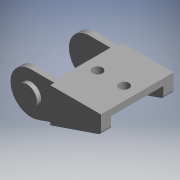
# Autodesk Inventor part: 045-16-2_se08f
Saved by Autodesk Inventor 2017.3 (Build 213256000, 256)
## iProperties
Part Number: 045-16-2_se08f
Material: Generic
Catalog Web Link: www.cadenas.de
Description: 045-16 -1, 045-16-2, 108-_ _-1PZ, 108-_ _-2PZ, 114-_-1PZ, 114-_-2PZ, 117-_-1PZ, 117-_-2PZ, 200F-_-1PZ,200F-_-2PZ, 300F-_-1PZ, 300F-_-2PZ-Flanges for Cable Carriers
Vendor: MISUMI
Document SubType Name: Modeling
Designer: partserver
Manufacturer: MISUMI
Mass: 1.82099 g
Surface Area: 19.911 cm^2
Volume: 1.82099 cm^3
Density: 1 g/cm^3
Appearance: PSOLRGB-192-192-192
Category: PARTsolutions
Company: MISUMI
Title: 045-16-2_se08f
Author: Cadenas PARTsolutions
Comments: Flanges for Cable Carriers
PSOL_IDENT_0: {$CADENAS_DATA\23d-libs\misumi\metric\07_slide_rails\se200f\se08f_body.prj},305 {VTYP=3D},{NB=045-16
PSOL_IDENT_1: -2_se08f},{LINA=045-16-2_se08f},{NN=045-16 -1, 045-16-2, 108-_ _-1PZ, 108-_ _-2PZ, 114-_-1PZ, 114-_-
PSOL_IDENT_2: 2PZ, 117-_-1PZ, 117-_-2PZ, 200F-_-1PZ,200F-_-2PZ, 300F-_-1PZ, 300F-_-2PZ},{DATE=30.06.2021 12:54:06}
PSOL_IDENT_3: ,{GEOMDATE=20.09.2012 00:00:00},{VERSION=},{LINEID=70},{WBVAR=NO,TS},{WBNUMERIC=NO}  {NB=045-16-2_se
PSOL_IDENT_4: 08f},{LINA=045-16-2_se08f},{KT=DUMMY},{PN=045-16-2},{TYPE=045-16},{TYS=045},{NO=16},{TS=2},{MAT=Spec
PSOL_IDENT_5: ial Plastic},{OT=-30~100},{NO0=16},{TS1= '1','For Free End', '2','For Fixed End' },{ACCE=_E045-16},{
PSOL_IDENT_6: ACCI=_Z045-16},{A=0},{B=22.0},{NCT=0},{X=22.3},{Y=-6.25},{XY=0.5}
NB: 045-16-2_se08f
NN: 045-16 -1, 045-16-2, 108-_ _-1PZ, 108-_ _-2PZ, 114-_-1PZ, 114-_-2PZ, 117-_-1PZ, 117-_-2PZ, 200F-_-1PZ,200F-_-2PZ, 300F-_-1PZ, 300F-_-2PZ
NT: Flanges for Cable Carriers
NBSYN: $PN._se08f
LINA: 045-16-2_se08f
CATALOG: Misumi
PN: 045-16-2
TYS: 045
NO: 16
TS: For Fixed End
MAT: Special Plastic
OT: -30~100
ACCE: _E045-16
ACCI: _Z045-16
A: 0
B: 22
NCT: 0
SUPPLIER: MISUMI
ARTICLENO: 045-16-2_se08f
BOMINFO: 045-16-2_se08f
CREATOR: CADENAS GmbH
Autodesk Inventor part; units mm, degrees
sketch "Sketch_77" plane through (0, 0, 0) normal (0, 0, 1) x (1, 0, 0)
  line L0 (0, 7.9) -> (0, -7.9)
  line L1 (0, -7.9) -> (16, -7.9)
  line L2 (16, -7.9) -> (16, 7.9)
  line L3 (16, 7.9) -> (0, 7.9)
  circle A0 centre (12, 0) radius 1.5
  circle A1 centre (4, 0) radius 1.5
  constraints: 8 end point, 2 centre point
extrude "Extrusion1" add sketch "Sketch_77" along normal blind 2
sketch "Sketch_78" plane through (0, 7.9, 0) normal (0, 1, 0) x (1, 0, 0)
  arc A0 (0, -4.5344) -> (0.6773, -5.4809) centre (1, -4.5344) ccw
  line L0 (0.6773, -5.4809) -> (20.283, -12.1656)
  arc A1 (20.283, -12.1656) -> (22.3, 0) centre (22.3, -6.25) ccw
  line L1 (22.3, 0) -> (0, 0)
  line L2 (0, 0) -> (0, -4.5344)
  constraints: 6 end point, 4 point on circle, 2 centre point
extrude "Extrusion2" add sketch "Sketch_78" along normal blind 1.85
sketch "Sketch_79" plane through (0, -7.9, 0) normal (0, 1, 0) x (1, 0, 0)
  arc A0 (0, -4.5344) -> (0.6773, -5.4809) centre (1, -4.5344) ccw
  line L0 (0.6773, -5.4809) -> (20.283, -12.1656)
  arc A1 (20.283, -12.1656) -> (22.3, 0) centre (22.3, -6.25) ccw
  line L1 (22.3, 0) -> (0, 0)
  line L2 (0, 0) -> (0, -4.5344)
  constraints: 6 end point, 4 point on circle, 2 centre point
extrude "Extrusion3" add sketch "Sketch_79" against normal blind 1.85
sketch "Sketch_80" plane through (0, 9.6, 0) normal (0, 1, 0) x (1, 0, 0)
  circle A0 centre (22.3, -6.25) radius 3
  constraints: 1 centre point
extrude "Extrusion4" add sketch "Sketch_80" along normal blind 1.4
sketch "Sketch_81" plane through (0, -9.6, 0) normal (0, 1, 0) x (1, 0, 0)
  circle A0 centre (22.3, -6.25) radius 3
  constraints: 1 centre point
extrude "Extrusion5" add sketch "Sketch_81" along normal mid plane 2.8
sketch "Sketch_82" plane through (0, 9.6, 0) normal (0, 1, 0) x (1, 0, 0)
  arc A0 (0, -4.5344) -> (0.6773, -5.4809) centre (1, -4.5344) ccw
  line L0 (0.6773, -5.4809) -> (15.3, -10.4666)
  line L1 (15.3, -10.4666) -> (15.3, 0)
  line L2 (15.3, 0) -> (0, 0)
  line L3 (0, 0) -> (0, -4.5344)
  constraints: 8 end point, 2 point on circle, 1 centre point
extrude "Extrusion6" add sketch "Sketch_82" along normal blind 1.4
sketch "Sketch_83" plane through (0, -9.6, 0) normal (0, 1, 0) x (1, 0, 0)
  arc A0 (0, -4.5344) -> (0.6773, -5.4809) centre (1, -4.5344) ccw
  line L0 (0.6773, -5.4809) -> (15.3, -10.4666)
  line L1 (15.3, -10.4666) -> (15.3, 0)
  line L2 (15.3, 0) -> (0, 0)
  line L3 (0, 0) -> (0, -4.5344)
  constraints: 8 end point, 2 point on circle, 1 centre point
extrude "Extrusion7" add sketch "Sketch_83" along normal mid plane 2.8
ref_plane "end_2_XY" through (22.3, 10.5, 6.25) normal (0, 1, 0) x (1, 0, 0)
ref_plane "end_2_YZ" through (22.3, 10.5, 6.25) normal (1, 0, 0) x (0, 0, -1)
ref_plane "end_2_ZX" through (22.3, 10.5, 6.25) normal (0, 0, -1) x (0, 1, 0)
ref_plane "end_move_XY" through (22.3, -11.5, 6.25) normal (0, -1, 0) x (1, 0, 0)
ref_plane "end_move_YZ" through (22.3, -11.5, 6.25) normal (1, 0, 0) x (0, 0, 1)
ref_plane "end_move_ZX" through (22.3, -11.5, 6.25) normal (0, 0, 1) x (0, -1, 0)
ref_plane "to_dummy_XY" through (0, 0, 0) normal (0, 0, 1) x (1, 0, 0)
ref_plane "to_dummy_YZ" through (0, 0, 0) normal (1, 0, 0) x (0, 1, 0)
ref_plane "to_dummy_ZX" through (0, 0, 0) normal (0, 1, 0) x (0, 0, 1)
body "Solid1"
